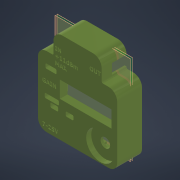
# Autodesk Inventor part: shell
Saved by Autodesk Inventor 2022 (Build 260153000, 153)
## iProperties
Created: 2021-12-11
Part Number: shell
Material: ABS Plastic
Document SubType Name: Modeling
Designer: nebst
Density: 1.06 g/cm^3
Appearance: Dark Olive
Author: nebst
Autodesk Inventor part; units mm, degrees
(part 1 of 2)
ref_plane "YZ Plane" through (0, 0, 0) normal (1, 0, 0) x (0, 1, 0)
ref_plane "XZ Plane" through (0, 0, 0) normal (0, 1, 0) x (-1, 0, 0)
ref_plane "XY Plane" through (0, 0, 0) normal (0, 0, 1) x (1, 0, 0)
ref_plane "board backside" through (0, 0, -1.6) normal (0, 0, -1) x (-1, 0, 0)
sketch "Sketch1" plane through (0, 0, -1.6) normal (0, 0, -1) x (-1, 0, 0)
  line L0 (-26.924, -27.6401) -> (-26.924, 15.0319) projected
  arc A0 (-26.924, -27.6401) -> (-24.384, -30.1801) centre (-24.384, -27.6401) ccw projected
  line L1 (24.384, -30.1801) -> (-24.384, -30.1801) projected
  arc A1 (24.384, -30.1801) -> (26.924, -27.6401) centre (24.384, -27.6401) ccw projected
  line L2 (26.924, 16.5559) -> (26.924, -27.6401) projected
  arc A2 (26.924, 16.5559) -> (24.384, 19.0959) centre (24.384, 16.5559) ccw projected
  line L3 (19.812, 19.0959) -> (24.384, 19.0959) projected
  arc A3 (17.272, 21.6359) -> (19.812, 19.0959) centre (19.812, 21.6359) ccw projected
  line L4 (17.272, 30.7799) -> (17.272, 21.6359) projected
  arc A4 (17.272, 30.7799) -> (14.732, 33.3199) centre (14.732, 30.7799) ccw projected
  line L5 (-14.732, 33.3199) -> (14.732, 33.3199) projected
  arc A5 (-14.732, 33.3199) -> (-17.272, 30.7799) centre (-14.732, 30.7799) ccw projected
  line L6 (-17.272, 21.6359) -> (-17.272, 30.7799) projected
  arc A6 (-19.812, 19.0959) -> (-17.272, 21.6359) centre (-19.812, 21.6359) ccw projected
  line L7 (-24.384, 19.0959) -> (-19.812, 19.0959) projected
  arc A7 (-24.384, 19.0959) -> (-26.924, 16.5559) centre (-24.384, 16.5559) ccw projected
  line L8 (-26.924, 15.0319) -> (-26.924, 16.5559) projected
  line L9 (20.978, -21.5601) -> (20.978, -23.5601) projected
  arc A8 (19.978, -23.5601) -> (20.978, -23.5601) centre (20.478, -23.5601) ccw projected
  line L10 (19.978, -23.5601) -> (19.978, -21.5601) projected
  arc A9 (20.978, -21.5601) -> (19.978, -21.5601) centre (20.478, -21.5601) ccw projected
  line L11 (16.478, -26.7601) -> (18.478, -26.7601) projected
  arc A10 (18.478, -27.7601) -> (18.478, -26.7601) centre (18.478, -27.2601) ccw projected
  line L12 (18.478, -27.7601) -> (16.478, -27.7601) projected
  arc A11 (16.478, -26.7601) -> (16.478, -27.7601) centre (16.478, -27.2601) ccw projected
  line L13 (14.978, -21.5601) -> (14.978, -23.5601) projected
  arc A12 (13.978, -23.5601) -> (14.978, -23.5601) centre (14.478, -23.5601) ccw projected
  line L14 (13.978, -23.5601) -> (13.978, -21.5601) projected
  arc A13 (14.978, -21.5601) -> (13.978, -21.5601) centre (14.478, -21.5601) ccw projected
  circle A14 centre (19.558, -14.3051) radius 0.5 projected
  circle A15 centre (24.003, -9.8601) radius 0.5 projected
  circle A16 centre (21.463, -9.8601) radius 0.5 projected
  circle A17 centre (18.923, -9.8601) radius 0.5 projected
  circle A18 centre (17.018, -14.3051) radius 0.5 projected
  circle A19 centre (16.383, -9.8601) radius 0.5 projected
  circle A20 centre (7.493, -14.3051) radius 0.5 projected
  circle A21 centre (4.953, -14.3051) radius 0.5 projected
  circle A22 centre (10.922, -1.2241) radius 0.5 projected
  circle A23 centre (8.382, -1.2241) radius 0.5 projected
  circle A24 centre (2.54, -5.0341) radius 0.35 projected
  circle A25 centre (0, -5.0341) radius 0.35 projected
  circle A26 centre (-10.287, -25.0201) radius 0.5 projected
  circle A27 centre (-10.287, -22.5201) radius 0.5 projected
  circle A28 centre (-10.287, -20.0201) radius 0.5 projected
  circle A29 centre (-17.787, -28.1201) radius 1.3 projected
  circle A30 centre (-24.787, -25.0201) radius 0.5 projected
  circle A31 centre (-17.787, -16.9201) radius 1.3 projected
  circle A32 centre (-24.787, -20.0201) radius 0.5 projected
  circle A33 centre (-2.54, -5.0341) radius 0.35 projected
  circle A34 centre (-5.08, -5.0341) radius 0.35 projected
  circle A35 centre (-7.62, -5.0341) radius 0.35 projected
  circle A36 centre (-10.16, -5.0341) radius 0.35 projected
  circle A37 centre (-12.7, -5.0341) radius 0.35 projected
  circle A38 centre (-15.24, -5.0341) radius 0.35 projected
  circle A39 centre (23.368, 10.4599) radius 0.5 projected
  circle A40 centre (20.828, 10.4599) radius 0.5 projected
  circle A41 centre (18.288, 10.4599) radius 0.5 projected
  circle A42 centre (10.922, 1.3159) radius 0.5 projected
  circle A43 centre (8.382, 1.3159) radius 0.5 projected
  circle A44 centre (10.922, 3.8559) radius 0.5 projected
  circle A45 centre (10.922, 6.3959) radius 0.5 projected
  circle A46 centre (8.382, 3.8559) radius 0.5 projected
  circle A47 centre (8.382, 6.3959) radius 0.5 projected
  circle A48 centre (2.54, 5.1259) radius 0.35 projected
  circle A49 centre (0, 5.1259) radius 0.35 projected
  circle A50 centre (16.818, 23.0329) radius 0.1 projected
  circle A51 centre (16.818, 23.6679) radius 0.1 projected
  circle A52 centre (16.31, 23.0329) radius 0.1 projected
  circle A53 centre (15.802, 23.0329) radius 0.1 projected
  circle A54 centre (15.294, 23.0329) radius 0.1 projected
  circle A55 centre (16.31, 23.6679) radius 0.1 projected
  circle A56 centre (15.802, 23.6679) radius 0.1 projected
  circle A57 centre (15.294, 23.6679) radius 0.1 projected
  circle A58 centre (14.786, 23.0329) radius 0.1 projected
  circle A59 centre (14.278, 23.0329) radius 0.1 projected
  circle A60 centre (13.77, 23.0329) radius 0.1 projected
  circle A61 centre (14.786, 23.6679) radius 0.1 projected
  circle A62 centre (14.278, 23.6679) radius 0.1 projected
  circle A63 centre (13.77, 23.6679) radius 0.1 projected
  circle A64 centre (13.262, 23.0329) radius 0.1 projected
  circle A65 centre (13.262, 23.6679) radius 0.1 projected
  circle A66 centre (16.818, 28.7479) radius 0.1 projected
  circle A67 centre (16.818, 29.3829) radius 0.1 projected
  circle A68 centre (16.31, 28.7479) radius 0.1 projected
  circle A69 centre (16.31, 29.3829) radius 0.1 projected
  circle A70 centre (15.802, 28.7479) radius 0.1 projected
  circle A71 centre (15.294, 28.7479) radius 0.1 projected
  circle A72 centre (15.802, 29.3829) radius 0.1 projected
  circle A73 centre (15.294, 29.3829) radius 0.1 projected
  circle A74 centre (14.786, 28.7479) radius 0.1 projected
  circle A75 centre (14.786, 29.3829) radius 0.1 projected
  circle A76 centre (14.278, 28.7479) radius 0.1 projected
  circle A77 centre (13.77, 28.7479) radius 0.1 projected
  circle A78 centre (14.278, 29.3829) radius 0.1 projected
  circle A79 centre (13.77, 29.3829) radius 0.1 projected
  circle A80 centre (13.262, 28.7479) radius 0.1 projected
  circle A81 centre (13.262, 29.3829) radius 0.1 projected
  circle A82 centre (1.508, 24.9539) radius 0.1 projected
  circle A83 centre (0.508, 24.9539) radius 0.1 projected
  circle A84 centre (1.508, 25.9539) radius 0.1 projected
  circle A85 centre (1.508, 26.9539) radius 0.1 projected
  circle A86 centre (0.508, 25.9539) radius 0.1 projected
  circle A87 centre (0.508, 26.9539) radius 0.1 projected
  circle A88 centre (-2.54, 5.1259) radius 0.35 projected
  circle A89 centre (-5.08, 5.1259) radius 0.35 projected
  circle A90 centre (-7.62, 5.1259) radius 0.35 projected
  circle A91 centre (-10.16, 5.1259) radius 0.35 projected
  circle A92 centre (-12.7, 5.1259) radius 0.35 projected
  circle A93 centre (-15.24, 5.1259) radius 0.35 projected
  circle A94 centre (-0.492, 24.9539) radius 0.1 projected
  circle A95 centre (-0.492, 25.9539) radius 0.1 projected
  circle A96 centre (-0.492, 26.9539) radius 0.1 projected
  circle A97 centre (-13.462, 23.0329) radius 0.1 projected
  circle A98 centre (-13.97, 23.0329) radius 0.1 projected
  circle A99 centre (-13.462, 23.6679) radius 0.1 projected
  circle A100 centre (-13.97, 23.6679) radius 0.1 projected
  circle A101 centre (-14.478, 23.0329) radius 0.1 projected
  circle A102 centre (-14.986, 23.0329) radius 0.1 projected
  circle A103 centre (-15.494, 23.0329) radius 0.1 projected
  circle A104 centre (-14.478, 23.6679) radius 0.1 projected
  circle A105 centre (-14.986, 23.6679) radius 0.1 projected
  circle A106 centre (-15.494, 23.6679) radius 0.1 projected
  circle A107 centre (-16.002, 23.0329) radius 0.1 projected
  circle A108 centre (-16.51, 23.0329) radius 0.1 projected
  circle A109 centre (-17.018, 23.0329) radius 0.1 projected
  circle A110 centre (-16.002, 23.6679) radius 0.1 projected
  circle A111 centre (-16.51, 23.6679) radius 0.1 projected
  circle A112 centre (-17.018, 23.6679) radius 0.1 projected
  circle A113 centre (-13.462, 28.7479) radius 0.1 projected
  circle A114 centre (-13.462, 29.3829) radius 0.1 projected
  circle A115 centre (-13.97, 28.7479) radius 0.1 projected
  circle A116 centre (-13.97, 29.3829) radius 0.1 projected
  circle A117 centre (-14.478, 28.7479) radius 0.1 projected
  circle A118 centre (-14.986, 28.7479) radius 0.1 projected
  circle A119 centre (-14.478, 29.3829) radius 0.1 projected
  circle A120 centre (-14.986, 29.3829) radius 0.1 projected
  circle A121 centre (-15.494, 28.7479) radius 0.1 projected
  circle A122 centre (-15.494, 29.3829) radius 0.1 projected
  circle A123 centre (-16.002, 28.7479) radius 0.1 projected
  circle A124 centre (-16.51, 28.7479) radius 0.1 projected
  circle A125 centre (-16.002, 29.3829) radius 0.1 projected
  circle A126 centre (-16.51, 29.3829) radius 0.1 projected
  circle A127 centre (-17.018, 28.7479) radius 0.1 projected
  circle A128 centre (-17.018, 29.3829) radius 0.1 projected
  line L15 (-27.074, 15.0319) -> (-27.074, -27.6401)
  arc A129 (-27.074, -27.6401) -> (-24.384, -30.3301) centre (-24.384, -27.6401) ccw
  line L16 (-24.384, -30.3301) -> (24.384, -30.3301)
  arc A130 (24.384, -30.3301) -> (27.074, -27.6401) centre (24.384, -27.6401) ccw
  line L17 (27.074, -27.6401) -> (27.074, 16.5559)
  arc A131 (27.074, 16.5559) -> (24.384, 19.2459) centre (24.384, 16.5559) ccw
  line L18 (24.384, 19.2459) -> (19.812, 19.2459)
  arc A132 (17.422, 21.6359) -> (19.812, 19.2459) centre (19.812, 21.6359) ccw
  line L19 (17.422, 21.6359) -> (17.422, 30.7799)
  arc A133 (17.422, 30.7799) -> (14.732, 33.4699) centre (14.732, 30.7799) ccw
  line L20 (14.732, 33.4699) -> (-14.732, 33.4699)
  arc A134 (-14.732, 33.4699) -> (-17.422, 30.7799) centre (-14.732, 30.7799) ccw
  line L21 (-17.422, 30.7799) -> (-17.422, 21.6359)
  arc A135 (-19.812, 19.2459) -> (-17.422, 21.6359) centre (-19.812, 21.6359) ccw
  line L22 (-19.812, 19.2459) -> (-24.384, 19.2459)
  arc A136 (-24.384, 19.2459) -> (-27.074, 16.5559) centre (-24.384, 16.5559) ccw
  line L23 (-27.074, 16.5559) -> (-27.074, 15.0319)
  line L24 (31.074, 13.9559) -> (31.074, -27.6401)
  arc A137 (24.384, -34.3301) -> (31.074, -27.6401) centre (24.384, -27.6401) ccw
  line L25 (24.384, -34.3301) -> (-24.384, -34.3301)
  arc A138 (-31.074, -27.6401) -> (-24.384, -34.3301) centre (-24.384, -27.6401) ccw
  line L26 (-31.074, -27.6401) -> (-31.074, 13.9559)
  line L27 (-18.922, 21.7459) -> (-18.922, 30.6799)
  line L28 (-12.132, 37.4699) -> (12.132, 37.4699)
  line L29 (18.922, 30.6799) -> (18.922, 21.7459)
  line L30 (19.922, 20.7459) -> (24.284, 20.7459)
  line L31 (-24.284, 20.7459) -> (-19.922, 20.7459)
  arc A139 (-24.284, 20.7459) -> (-31.074, 13.9559) centre (-24.284, 13.9559) ccw
  arc A140 (31.074, 13.9559) -> (24.284, 20.7459) centre (24.284, 13.9559) ccw
  arc A141 (-19.922, 20.7459) -> (-18.922, 21.7459) centre (-19.922, 21.7459) ccw
  arc A142 (18.922, 21.7459) -> (19.922, 20.7459) centre (19.922, 21.7459) ccw
  arc A143 (18.922, 30.6799) -> (12.132, 37.4699) centre (12.132, 30.6799) ccw
  arc A144 (-12.132, 37.4699) -> (-18.922, 30.6799) centre (-12.132, 30.6799) ccw
  point P0 (0, 0)
  dimension "d0" = 0.15
  dimension "d3" = 6.79
  dimension "d4" = 4
  dimension "d5" = 4
  dimension "d6" = 1
  dimension "d7" = 1.5
  dimension "d8" = 1.5
  dimension "d9" = 1.5
  dimension "d10" = 1.5
  dimension "d11" = 6.79
  constraints: 34 end point, 32 point on circle, 16 centre point, 12 tangent, 3 equal radius, 20 other
  measures "d0" distance between parallel lines of L0 L15
  measures "d3" radius of A139
  measures "d4" distance between parallel lines of L20 L28
  measures "d5" distance between parallel lines of L26 L15
  measures "d6" radius of A141
  measures "d7" distance between parallel lines of L18 L30
  measures "d8" distance between parallel lines of L22 L31
  measures "d9" distance between parallel lines of L21 L27
  measures "d10" distance between parallel lines of L19 L29
  measures "d11" radius of A143
extrude "side walls" add sketch "Sketch1" against normal blind 13.5 contours L24 A137 L25 A138 L26 A139 L31 A141 L27 A144 L28 A143 L29 A142 L30 A140
sketch "Sketch2" plane through (0, 0, 11.9) normal (0, 0, 1) x (1, 0, 0)
  line L0 (12.132, 37.4699) -> (-12.132, 37.4699)
  arc A0 (-12.132, 37.4699) -> (-18.922, 30.6799) centre (-12.132, 30.6799) ccw
  line L1 (-18.922, 30.6799) -> (-18.922, 21.7459)
  arc A1 (-19.922, 20.7459) -> (-18.922, 21.7459) centre (-19.922, 21.7459) ccw
  line L2 (-19.922, 20.7459) -> (-24.284, 20.7459)
  arc A2 (-24.284, 20.7459) -> (-31.074, 13.9559) centre (-24.284, 13.9559) ccw
  line L3 (-31.074, 13.9559) -> (-31.074, -27.6401)
  arc A3 (-31.074, -27.6401) -> (-24.384, -34.3301) centre (-24.384, -27.6401) ccw
  line L4 (-24.384, -34.3301) -> (24.384, -34.3301)
  arc A4 (24.384, -34.3301) -> (31.074, -27.6401) centre (24.384, -27.6401) ccw
  line L5 (31.074, -27.6401) -> (31.074, 13.9559)
  arc A5 (31.074, 13.9559) -> (24.284, 20.7459) centre (24.284, 13.9559) ccw
  line L6 (24.284, 20.7459) -> (19.922, 20.7459)
  arc A6 (18.922, 21.7459) -> (19.922, 20.7459) centre (19.922, 21.7459) ccw
  line L7 (18.922, 21.7459) -> (18.922, 30.6799)
  arc A7 (18.922, 30.6799) -> (12.132, 37.4699) centre (12.132, 30.6799) ccw
  arc A8 (17.422, 21.6359) -> (19.812, 19.2459) centre (19.812, 21.6359) ccw
  line L8 (19.812, 19.2459) -> (24.384, 19.2459)
  arc A9 (27.074, 16.5559) -> (24.384, 19.2459) centre (24.384, 16.5559) ccw
  line L9 (27.074, 16.5559) -> (27.074, -27.6401)
  arc A10 (24.384, -30.3301) -> (27.074, -27.6401) centre (24.384, -27.6401) ccw
  line L10 (24.384, -30.3301) -> (-24.384, -30.3301)
  arc A11 (-27.074, -27.6401) -> (-24.384, -30.3301) centre (-24.384, -27.6401) ccw
  line L11 (-27.074, -27.6401) -> (-27.074, 16.5559)
  arc A12 (-24.384, 19.2459) -> (-27.074, 16.5559) centre (-24.384, 16.5559) ccw
  line L12 (-24.384, 19.2459) -> (-19.812, 19.2459)
  arc A13 (-19.812, 19.2459) -> (-17.422, 21.6359) centre (-19.812, 21.6359) ccw
  line L13 (-17.422, 21.6359) -> (-17.422, 30.7799)
  arc A14 (-14.732, 33.4699) -> (-17.422, 30.7799) centre (-14.732, 30.7799) ccw
  line L14 (-14.732, 33.4699) -> (14.732, 33.4699)
  arc A15 (17.422, 30.7799) -> (14.732, 33.4699) centre (14.732, 30.7799) ccw
  line L15 (17.422, 30.7799) -> (17.422, 21.6359)
  line L16 (-24.638, 9.4439) -> (-24.384, 9.1899)
  line L17 (-24.384, 9.1899) -> (-22.352, 9.1899)
  line L18 (-22.352, 9.1899) -> (-22.098, 9.4439)
  line L19 (-22.098, 9.4439) -> (-21.844, 9.1899)
  line L20 (-21.844, 9.1899) -> (-19.812, 9.1899)
  line L21 (-19.812, 9.1899) -> (-19.558, 9.4439)
  line L22 (-19.558, 9.4439) -> (-19.304, 9.1899)
  line L23 (-19.304, 9.1899) -> (-17.272, 9.1899)
  line L24 (-17.272, 9.1899) -> (-17.018, 9.4439)
  line L25 (-17.018, 9.4439) -> (-17.018, 11.4759)
  line L26 (-17.018, 11.4759) -> (-17.272, 11.7299)
  line L27 (-17.272, 11.7299) -> (-19.304, 11.7299)
  line L28 (-19.304, 11.7299) -> (-19.558, 11.4759)
  line L29 (-19.558, 11.4759) -> (-19.812, 11.7299)
  line L30 (-19.812, 11.7299) -> (-21.844, 11.7299)
  line L31 (-21.844, 11.7299) -> (-22.098, 11.4759)
  line L32 (-22.098, 11.4759) -> (-22.352, 11.7299)
  line L33 (-22.352, 11.7299) -> (-24.384, 11.7299)
  line L34 (-24.384, 11.7299) -> (-24.638, 11.4759)
  line L35 (-24.638, 11.4759) -> (-24.638, 9.4439)
  line L36 (-23.048, 10.7799) -> (-23.688, 10.7799)
  line L37 (-23.048, 10.7799) -> (-23.048, 10.1399)
  line L38 (-23.048, 10.1399) -> (-23.688, 10.1399)
  line L39 (-23.688, 10.7799) -> (-23.688, 10.1399)
  line L40 (-20.508, 10.7799) -> (-20.508, 10.1399)
  line L41 (-20.508, 10.1399) -> (-21.148, 10.1399)
  line L42 (-21.148, 10.7799) -> (-21.148, 10.1399)
  line L43 (-20.508, 10.7799) -> (-21.148, 10.7799)
  line L44 (-18.608, 10.7799) -> (-18.608, 10.1399)
  line L45 (-17.968, 10.7799) -> (-18.608, 10.7799)
  line L46 (-17.968, 10.7799) -> (-17.968, 10.1399)
  line L47 (-17.968, 10.1399) -> (-18.608, 10.1399)
  line L48 (-15.113, -8.8441) -> (-15.367, -8.5901)
  line L49 (-15.367, -8.5901) -> (-17.399, -8.5901)
  line L50 (-17.399, -8.5901) -> (-17.653, -8.8441)
  line L51 (-17.653, -8.8441) -> (-17.907, -8.5901)
  line L52 (-17.907, -8.5901) -> (-19.939, -8.5901)
  line L53 (-19.939, -8.5901) -> (-20.193, -8.8441)
  line L54 (-20.193, -8.8441) -> (-20.447, -8.5901)
  line L55 (-20.447, -8.5901) -> (-22.479, -8.5901)
  line L56 (-22.479, -8.5901) -> (-22.733, -8.8441)
  line L57 (-22.733, -8.8441) -> (-22.987, -8.5901)
  line L58 (-22.987, -8.5901) -> (-25.019, -8.5901)
  line L59 (-25.019, -8.5901) -> (-25.273, -8.8441)
  line L60 (-25.273, -8.8441) -> (-25.273, -10.8761)
  line L61 (-25.273, -10.8761) -> (-25.019, -11.1301)
  line L62 (-25.019, -11.1301) -> (-22.987, -11.1301)
  line L63 (-22.987, -11.1301) -> (-22.733, -10.8761)
  line L64 (-22.733, -10.8761) -> (-22.479, -11.1301)
  line L65 (-22.479, -11.1301) -> (-20.447, -11.1301)
  line L66 (-20.447, -11.1301) -> (-20.193, -10.8761)
  line L67 (-20.193, -10.8761) -> (-19.939, -11.1301)
  line L68 (-19.939, -11.1301) -> (-17.907, -11.1301)
  line L69 (-17.907, -11.1301) -> (-17.653, -10.8761)
  line L70 (-17.653, -10.8761) -> (-17.399, -11.1301)
  line L71 (-17.399, -11.1301) -> (-15.367, -11.1301)
  line L72 (-15.367, -11.1301) -> (-15.113, -10.8761)
  line L73 (-15.113, -10.8761) -> (-15.113, -8.8441)
  line L74 (-21.143, -10.1801) -> (-21.143, -9.5401)
  line L75 (-21.783, -10.1801) -> (-21.143, -10.1801)
  line L76 (-21.783, -10.1801) -> (-21.783, -9.5401)
  line L77 (-21.783, -9.5401) -> (-21.143, -9.5401)
  line L78 (-24.323, -10.1801) -> (-23.683, -10.1801)
  line L79 (-24.323, -10.1801) -> (-24.323, -9.5401)
  line L80 (-24.323, -9.5401) -> (-23.683, -9.5401)
  line L81 (-23.683, -10.1801) -> (-23.683, -9.5401)
  line L82 (-16.703, -10.1801) -> (-16.063, -10.1801)
  line L83 (-16.703, -10.1801) -> (-16.703, -9.5401)
  line L84 (-16.703, -9.5401) -> (-16.063, -9.5401)
  line L85 (-16.063, -10.1801) -> (-16.063, -9.5401)
  line L86 (-18.603, -10.1801) -> (-18.603, -9.5401)
  line L87 (-19.243, -10.1801) -> (-18.603, -10.1801)
  line L88 (-19.243, -10.1801) -> (-19.243, -9.5401)
  line L89 (-19.243, -9.5401) -> (-18.603, -9.5401)
  line L90 (-15.748, -13.2891) -> (-16.002, -13.0351)
  line L91 (-16.002, -13.0351) -> (-18.034, -13.0351)
  line L92 (-18.034, -13.0351) -> (-18.288, -13.2891)
  line L93 (-18.288, -13.2891) -> (-18.542, -13.0351)
  line L94 (-18.542, -13.0351) -> (-20.574, -13.0351)
  line L95 (-20.574, -13.0351) -> (-20.828, -13.2891)
  line L96 (-20.828, -13.2891) -> (-20.828, -15.3211)
  line L97 (-20.828, -15.3211) -> (-20.574, -15.5751)
  line L98 (-20.574, -15.5751) -> (-18.542, -15.5751)
  line L99 (-18.542, -15.5751) -> (-18.288, -15.3211)
  line L100 (-18.288, -15.3211) -> (-18.034, -15.5751)
  line L101 (-18.034, -15.5751) -> (-16.002, -15.5751)
  line L102 (-16.002, -15.5751) -> (-15.748, -15.3211)
  line L103 (-15.748, -15.3211) -> (-15.748, -13.2891)
  line L104 (-17.338, -14.6251) -> (-17.338, -13.9851)
  line L105 (-17.338, -13.9851) -> (-16.698, -13.9851)
  line L106 (-16.698, -14.6251) -> (-16.698, -13.9851)
  line L107 (-17.338, -14.6251) -> (-16.698, -14.6251)
  line L108 (-19.878, -14.6251) -> (-19.878, -13.9851)
  line L109 (-19.878, -13.9851) -> (-19.238, -13.9851)
  line L110 (-19.238, -14.6251) -> (-19.238, -13.9851)
  line L111 (-19.878, -14.6251) -> (-19.238, -14.6251)
  line L112 (-3.683, -13.2891) -> (-3.937, -13.0351)
  line L113 (-3.937, -13.0351) -> (-5.969, -13.0351)
  line L114 (-5.969, -13.0351) -> (-6.223, -13.2891)
  line L115 (-6.223, -13.2891) -> (-6.477, -13.0351)
  line L116 (-6.477, -13.0351) -> (-8.509, -13.0351)
  line L117 (-8.509, -13.0351) -> (-8.763, -13.2891)
  line L118 (-8.763, -13.2891) -> (-8.763, -15.3211)
  line L119 (-8.763, -15.3211) -> (-8.509, -15.5751)
  line L120 (-8.509, -15.5751) -> (-6.477, -15.5751)
  line L121 (-6.477, -15.5751) -> (-6.223, -15.3211)
  line L122 (-6.223, -15.3211) -> (-5.969, -15.5751)
  line L123 (-5.969, -15.5751) -> (-3.937, -15.5751)
  line L124 (-3.937, -15.5751) -> (-3.683, -15.3211)
  line L125 (-3.683, -15.3211) -> (-3.683, -13.2891)
  line L126 (-5.273, -14.6251) -> (-5.273, -13.9851)
  line L127 (-5.273, -13.9851) -> (-4.633, -13.9851)
  line L128 (-4.633, -14.6251) -> (-4.633, -13.9851)
  line L129 (-5.273, -14.6251) -> (-4.633, -14.6251)
  line L130 (-7.813, -14.6251) -> (-7.813, -13.9851)
  line L131 (-7.813, -13.9851) -> (-7.173, -13.9851)
  line L132 (-7.173, -14.6251) -> (-7.173, -13.9851)
  line L133 (-7.813, -14.6251) -> (-7.173, -14.6251)
  line L134 (26.4, -6.3041) -> (26.4, 6.3959)
  line L135 (26.4, 6.3959) -> (-13.7, 6.3959)
  line L136 (-13.7, 6.3959) -> (-13.7, -6.3041)
  line L137 (-13.7, -6.3041) -> (26.4, -6.3041)
  line L138 (20.3476, 4.1754) -> (19.9121, 4.7197)
  line L139 (19.9121, 4.7197) -> (20.3014, 5.0311)
  line L140 (20.3014, 5.0311) -> (24.5951, 5.0464)
  line L141 (24.5951, 5.0464) -> (24.8689, 4.7041)
  line L142 (24.8689, 4.7041) -> (24.208, 4.1754)
  line L143 (24.208, 4.1754) -> (20.3476, 4.1754)
  line L144 (24.6494, 0.1774) -> (23.8633, 0.6371)
  line L145 (23.8633, 0.6371) -> (24.387, 3.897)
  line L146 (24.387, 3.897) -> (25.052, 4.4753)
  line L147 (25.052, 4.4753) -> (25.2917, 4.1756)
  line L148 (25.2917, 4.1756) -> (24.6494, 0.1774)
  line L149 (19.3167, -0.5453) -> (18.793, -3.8051)
  line L150 (18.793, -3.8051) -> (18.128, -4.3835)
  line L151 (18.128, -4.3835) -> (17.8883, -4.0838)
  line L152 (17.8883, -4.0838) -> (18.5306, -0.0855)
  line L153 (18.5306, -0.0855) -> (19.3167, -0.5453)
  line L154 (23.2679, -4.6279) -> (22.8786, -4.9393)
  line L155 (22.8786, -4.9393) -> (18.5849, -4.9546)
  line L156 (18.5849, -4.9546) -> (18.3111, -4.6123)
  line L157 (18.3111, -4.6123) -> (18.972, -4.0835)
  line L158 (18.972, -4.0835) -> (22.8324, -4.0835)
  line L159 (22.8324, -4.0835) -> (23.2679, -4.6279)
  line L160 (14.892, 4.4753) -> (15.1317, 4.1756)
  line L161 (15.1317, 4.1756) -> (14.4894, 0.1774)
  line L162 (14.4894, 0.1774) -> (13.7033, 0.6371)
  line L163 (13.7033, 0.6371) -> (14.227, 3.897)
  line L164 (14.227, 3.897) -> (14.892, 4.4753)
  line L165 (12.6724, -4.0835) -> (13.1079, -4.6279)
  line L166 (13.1079, -4.6279) -> (12.7186, -4.9393)
  line L167 (12.7186, -4.9393) -> (8.4249, -4.9546)
  line L168 (8.4249, -4.9546) -> (8.1511, -4.6123)
  line L169 (8.1511, -4.6123) -> (8.812, -4.0835)
  line L170 (8.812, -4.0835) -> (12.6724, -4.0835)
  line L171 (8.3706, -0.0855) -> (9.1567, -0.5453)
  line L172 (9.1567, -0.5453) -> (8.633, -3.8051)
  line L173 (8.633, -3.8051) -> (7.968, -4.3835)
  line L174 (7.968, -4.3835) -> (7.7283, -4.0838)
  line L175 (7.7283, -4.0838) -> (8.3706, -0.0855)
  line L176 (14.7089, 4.7041) -> (14.048, 4.1754)
  line L177 (14.048, 4.1754) -> (10.1876, 4.1754)
  line L178 (10.1876, 4.1754) -> (9.7521, 4.7197)
  line L179 (9.7521, 4.7197) -> (10.1414, 5.0311)
  line L180 (10.1414, 5.0311) -> (14.4351, 5.0464)
  line L181 (14.4351, 5.0464) -> (14.7089, 4.7041)
  line L182 (4.732, 4.4753) -> (4.9717, 4.1756)
  line L183 (4.9717, 4.1756) -> (4.3294, 0.1774)
  line L184 (4.3294, 0.1774) -> (3.5433, 0.6371)
  line L185 (3.5433, 0.6371) -> (4.067, 3.897)
  line L186 (4.067, 3.897) -> (4.732, 4.4753)
  line L187 (2.5124, -4.0835) -> (2.9479, -4.6279)
  line L188 (2.9479, -4.6279) -> (2.5586, -4.9393)
  line L189 (2.5586, -4.9393) -> (-1.7351, -4.9546)
  line L190 (-1.7351, -4.9546) -> (-2.0089, -4.6123)
  line L191 (-2.0089, -4.6123) -> (-1.348, -4.0835)
  line L192 (-1.348, -4.0835) -> (2.5124, -4.0835)
  line L193 (-1.7894, -0.0855) -> (-1.0033, -0.5453)
  line L194 (-1.0033, -0.5453) -> (-1.527, -3.8051)
  line L195 (-1.527, -3.8051) -> (-2.192, -4.3835)
  line L196 (-2.192, -4.3835) -> (-2.4317, -4.0838)
  line L197 (-2.4317, -4.0838) -> (-1.7894, -0.0855)
  line L198 (4.5489, 4.7041) -> (3.888, 4.1754)
  line L199 (3.888, 4.1754) -> (0.0276, 4.1754)
  line L200 (0.0276, 4.1754) -> (-0.4079, 4.7197)
  line L201 (-0.4079, 4.7197) -> (-0.0186, 5.0311)
  line L202 (-0.0186, 5.0311) -> (4.2751, 5.0464)
  line L203 (4.2751, 5.0464) -> (4.5489, 4.7041)
  line L204 (-7.6476, -4.0835) -> (-7.2121, -4.6279)
  line L205 (-7.2121, -4.6279) -> (-7.6014, -4.9393)
  line L206 (-7.6014, -4.9393) -> (-11.8951, -4.9546)
  line L207 (-11.8951, -4.9546) -> (-12.1689, -4.6123)
  line L208 (-12.1689, -4.6123) -> (-11.508, -4.0835)
  line L209 (-11.508, -4.0835) -> (-7.6476, -4.0835)
  line L210 (-5.428, 4.4753) -> (-5.1883, 4.1756)
  line L211 (-5.1883, 4.1756) -> (-5.8306, 0.1774)
  line L212 (-5.8306, 0.1774) -> (-6.6167, 0.6371)
  line L213 (-6.6167, 0.6371) -> (-6.093, 3.897)
  line L214 (-6.093, 3.897) -> (-5.428, 4.4753)
  line L215 (-5.6111, 4.7041) -> (-6.272, 4.1754)
  line L216 (-6.272, 4.1754) -> (-10.1324, 4.1754)
  line L217 (-10.1324, 4.1754) -> (-10.5679, 4.7197)
  line L218 (-10.5679, 4.7197) -> (-10.1786, 5.0311)
  line L219 (-10.1786, 5.0311) -> (-5.8849, 5.0464)
  line L220 (-5.8849, 5.0464) -> (-5.6111, 4.7041)
  line L221 (-11.9494, -0.0855) -> (-11.1633, -0.5453)
  line L222 (-11.1633, -0.5453) -> (-11.687, -3.8051)
  line L223 (-11.687, -3.8051) -> (-12.352, -4.3835)
  line L224 (-12.352, -4.3835) -> (-12.5917, -4.0838)
  line L225 (-12.5917, -4.0838) -> (-11.9494, -0.0855)
  circle A16 centre (-5.5899, -4.3761) radius 0.6
  circle A17 centre (4.5701, -4.3761) radius 0.6
  circle A18 centre (14.7301, -4.3761) radius 0.6
  circle A19 centre (24.8901, -4.3761) radius 0.6
  circle A20 centre (5.9297, -2.4744) radius 0.6
  circle A21 centre (6.8216, 2.5384) radius 0.6
  circle A22 centre (17.784, 4.4351) radius 0.6221
  line L226 (-10.3651, 3.975) -> (-10.8347, 4.4753)
  line L227 (-10.9279, 0.6371) -> (-10.3651, 3.975)
  line L228 (-11.9471, 0.1774) -> (-10.9279, 0.6371)
  line L229 (-11.2468, 4.0885) -> (-11.9471, 0.1774)
  line L230 (-10.8347, 4.4753) -> (-11.2468, 4.0885)
  line L231 (-7.1965, -0.4291) -> (-6.2226, 0.0459)
  line L232 (-10.6853, -0.4291) -> (-7.1965, -0.4291)
  line L233 (-11.508, 0.0459) -> (-10.6853, -0.4291)
  line L234 (-11.508, 0.0459) -> (-10.5341, 0.5209)
  line L235 (-6.9453, 0.5209) -> (-10.5341, 0.5209)
  line L236 (-6.2226, 0.0459) -> (-6.9453, 0.5209)
  line L237 (-6.5332, -3.9967) -> (-5.8329, -0.0855)
  line L238 (-6.9453, -4.3835) -> (-6.5332, -3.9967)
  line L239 (-7.4149, -3.8831) -> (-6.9453, -4.3835)
  line L240 (-6.8521, -0.5453) -> (-7.4149, -3.8831)
  line L241 (-5.8329, -0.0855) -> (-6.8521, -0.5453)
  line L242 (2.9635, -0.4291) -> (3.9374, 0.0459)
  line L243 (-0.5253, -0.4291) -> (2.9635, -0.4291)
  line L244 (-1.348, 0.0459) -> (-0.5253, -0.4291)
  line L245 (-1.348, 0.0459) -> (-0.3741, 0.5209)
  line L246 (3.2147, 0.5209) -> (-0.3741, 0.5209)
  line L247 (3.9374, 0.0459) -> (3.2147, 0.5209)
  line L248 (-0.2051, 3.975) -> (-0.6747, 4.4753)
  line L249 (-0.7679, 0.6371) -> (-0.2051, 3.975)
  line L250 (-1.7871, 0.1774) -> (-0.7679, 0.6371)
  line L251 (-1.0868, 4.0885) -> (-1.7871, 0.1774)
  line L252 (-0.6747, 4.4753) -> (-1.0868, 4.0885)
  line L253 (3.6268, -3.9967) -> (4.3271, -0.0855)
  line L254 (3.2147, -4.3835) -> (3.6268, -3.9967)
  line L255 (2.7451, -3.8831) -> (3.2147, -4.3835)
  line L256 (3.3079, -0.5453) -> (2.7451, -3.8831)
  line L257 (4.3271, -0.0855) -> (3.3079, -0.5453)
  line L258 (9.9549, 3.975) -> (9.4853, 4.4753)
  line L259 (9.3921, 0.6371) -> (9.9549, 3.975)
  line L260 (8.3729, 0.1774) -> (9.3921, 0.6371)
  line L261 (9.0732, 4.0885) -> (8.3729, 0.1774)
  line L262 (9.4853, 4.4753) -> (9.0732, 4.0885)
  line L263 (13.7868, -3.9967) -> (14.4871, -0.0855)
  line L264 (13.3747, -4.3835) -> (13.7868, -3.9967)
  line L265 (12.9051, -3.8831) -> (13.3747, -4.3835)
  line L266 (13.4679, -0.5453) -> (12.9051, -3.8831)
  line L267 (14.4871, -0.0855) -> (13.4679, -0.5453)
  line L268 (13.1235, -0.4291) -> (14.0974, 0.0459)
  line L269 (9.6347, -0.4291) -> (13.1235, -0.4291)
  line L270 (8.812, 0.0459) -> (9.6347, -0.4291)
  line L271 (8.812, 0.0459) -> (9.7859, 0.5209)
  line L272 (13.3747, 0.5209) -> (9.7859, 0.5209)
  line L273 (14.0974, 0.0459) -> (13.3747, 0.5209)
  line L274 (19.2332, 4.0885) -> (18.5329, 0.1774)
  line L275 (19.6453, 4.4753) -> (19.2332, 4.0885)
  line L276 (20.1149, 3.975) -> (19.6453, 4.4753)
  line L277 (19.5521, 0.6371) -> (20.1149, 3.975)
  line L278 (18.5329, 0.1774) -> (19.5521, 0.6371)
  line L279 (24.6471, -0.0855) -> (23.6279, -0.5453)
  line L280 (23.9468, -3.9967) -> (24.6471, -0.0855)
  line L281 (23.5347, -4.3835) -> (23.9468, -3.9967)
  line L282 (23.0651, -3.8831) -> (23.5347, -4.3835)
  line L283 (23.6279, -0.5453) -> (23.0651, -3.8831)
  line L284 (24.2574, 0.0459) -> (23.5347, 0.5209)
  line L285 (23.2835, -0.4291) -> (24.2574, 0.0459)
  line L286 (19.7947, -0.4291) -> (23.2835, -0.4291)
  line L287 (18.972, 0.0459) -> (19.7947, -0.4291)
  line L288 (18.972, 0.0459) -> (19.9459, 0.5209)
  line L289 (23.5347, 0.5209) -> (19.9459, 0.5209)
  line L290 (-22.0511, 12.2299) -> (-19.6049, 12.2299)
  line L291 (-19.6049, 12.2299) -> (-19.558, 12.183)
  line L292 (-19.558, 12.183) -> (-19.5111, 12.2299)
  line L293 (-19.5111, 12.2299) -> (-17.0649, 12.2299)
  line L294 (-17.0649, 12.2299) -> (-16.518, 11.683)
  line L295 (-16.518, 11.683) -> (-16.518, 9.2368)
  line L296 (-16.518, 9.2368) -> (-17.0649, 8.6899)
  line L297 (-17.0649, 8.6899) -> (-19.5111, 8.6899)
  line L298 (-19.5111, 8.6899) -> (-19.558, 8.7368)
  line L299 (-19.558, 8.7368) -> (-19.6049, 8.6899)
  line L300 (-19.6049, 8.6899) -> (-22.0511, 8.6899)
  line L301 (-22.0511, 8.6899) -> (-22.098, 8.7368)
  line L302 (-22.098, 8.7368) -> (-22.1449, 8.6899)
  line L303 (-22.1449, 8.6899) -> (-24.5911, 8.6899)
  line L304 (-24.5911, 8.6899) -> (-25.138, 9.2368)
  line L305 (-25.138, 9.2368) -> (-25.138, 11.683)
  line L306 (-25.138, 11.683) -> (-24.5911, 12.2299)
  line L307 (-24.5911, 12.2299) -> (-22.1449, 12.2299)
  line L308 (-22.1449, 12.2299) -> (-22.098, 12.183)
  line L309 (-22.098, 12.183) -> (-22.0511, 12.2299)
  line L310 (-13.9, 6.5959) -> (26.6, 6.5959)
  line L311 (26.6, 6.5959) -> (26.6, -6.5041)
  line L312 (26.6, -6.5041) -> (-13.9, -6.5041)
  line L313 (-13.9, -6.5041) -> (-13.9, 6.5959)
  line L314 (-20.1461, -8.0901) -> (-17.6999, -8.0901)
  line L315 (-17.6999, -8.0901) -> (-17.653, -8.137)
  line L316 (-17.653, -8.137) -> (-17.6061, -8.0901)
  line L317 (-17.6061, -8.0901) -> (-15.1599, -8.0901)
  line L318 (-15.1599, -8.0901) -> (-14.613, -8.637)
  line L319 (-14.613, -8.637) -> (-14.613, -11.0832)
  line L320 (-14.613, -11.0832) -> (-15.1599, -11.6301)
  line L321 (-15.1599, -11.6301) -> (-17.6061, -11.6301)
  line L322 (-17.6061, -11.6301) -> (-17.653, -11.5832)
  line L323 (-17.653, -11.5832) -> (-17.6999, -11.6301)
  line L324 (-17.6999, -11.6301) -> (-20.1461, -11.6301)
  line L325 (-20.1461, -11.6301) -> (-20.193, -11.5832)
  line L326 (-20.193, -11.5832) -> (-20.2399, -11.6301)
  line L327 (-20.2399, -11.6301) -> (-22.6861, -11.6301)
  line L328 (-22.6861, -11.6301) -> (-22.733, -11.5832)
  line L329 (-22.733, -11.5832) -> (-22.7799, -11.6301)
  line L330 (-22.7799, -11.6301) -> (-25.2261, -11.6301)
  line L331 (-25.2261, -11.6301) -> (-25.773, -11.0832)
  line L332 (-25.773, -11.0832) -> (-25.773, -8.637)
  line L333 (-25.773, -8.637) -> (-25.2261, -8.0901)
  line L334 (-25.2261, -8.0901) -> (-22.7799, -8.0901)
  line L335 (-22.7799, -8.0901) -> (-22.733, -8.137)
  line L336 (-22.733, -8.137) -> (-22.6861, -8.0901)
  line L337 (-22.6861, -8.0901) -> (-20.2399, -8.0901)
  line L338 (-20.2399, -8.0901) -> (-20.193, -8.137)
  line L339 (-20.193, -8.137) -> (-20.1461, -8.0901)
  line L340 (-20.7811, -12.5351) -> (-18.3349, -12.5351)
  line L341 (-18.3349, -12.5351) -> (-18.288, -12.582)
  line L342 (-18.288, -12.582) -> (-18.2411, -12.5351)
  line L343 (-18.2411, -12.5351) -> (-15.7949, -12.5351)
  line L344 (-15.7949, -12.5351) -> (-15.248, -13.082)
  line L345 (-15.248, -13.082) -> (-15.248, -15.5282)
  line L346 (-15.248, -15.5282) -> (-15.7949, -16.0751)
  line L347 (-15.7949, -16.0751) -> (-18.2411, -16.0751)
  line L348 (-18.2411, -16.0751) -> (-18.288, -16.0282)
  line L349 (-18.288, -16.0282) -> (-18.3349, -16.0751)
  line L350 (-18.3349, -16.0751) -> (-20.7811, -16.0751)
  line L351 (-20.7811, -16.0751) -> (-21.328, -15.5282)
  line L352 (-21.328, -15.5282) -> (-21.328, -13.082)
  line L353 (-21.328, -13.082) -> (-20.7811, -12.5351)
  line L354 (-8.7161, -12.5351) -> (-6.2699, -12.5351)
  line L355 (-6.2699, -12.5351) -> (-6.223, -12.582)
  line L356 (-6.223, -12.582) -> (-6.1761, -12.5351)
  line L357 (-6.1761, -12.5351) -> (-3.7299, -12.5351)
  line L358 (-3.7299, -12.5351) -> (-3.183, -13.082)
  line L359 (-3.183, -13.082) -> (-3.183, -15.5282)
  line L360 (-3.183, -15.5282) -> (-3.7299, -16.0751)
  line L361 (-3.7299, -16.0751) -> (-6.1761, -16.0751)
  line L362 (-6.1761, -16.0751) -> (-6.223, -16.0282)
  line L363 (-6.223, -16.0282) -> (-6.2699, -16.0751)
  line L364 (-6.2699, -16.0751) -> (-8.7161, -16.0751)
  line L365 (-8.7161, -16.0751) -> (-9.263, -15.5282)
  line L366 (-9.263, -15.5282) -> (-9.263, -13.082)
  line L367 (-9.263, -13.082) -> (-8.7161, -12.5351)
  circle A23 centre (17.787, -22.5201) radius 1.5
  circle A24 centre (17.787, -22.5201) radius 3.75
  point P0 (0, 0)
extrude "front cutouts" add sketch "Sketch2" against normal blind 6 contours A8 L8 A9 L9 A10 L10 A11 L11 A12 L12 A13 L13 A14 L14 A15 L15
sketch "Sketch3" plane through (0, 0, -1.6) normal (0, 0, -1) x (-1, 0, 0)
  line L0 (-9.387, -15.4201) -> (-25.487, -15.4201)
  line L1 (-25.487, -15.4201) -> (-25.487, -26.6701)
  line L2 (-22.487, -29.6701) -> (-9.387, -29.6701)
  line L3 (-9.387, -29.6701) -> (-9.387, -15.4201)
  line L4 (-15.077, -28.4201) -> (-13.287, -28.4201) projected
  line L5 (-13.287, -16.6201) -> (-15.077, -16.6201) projected
  line L6 (-11.787, -18.5201) -> (-11.787, -26.5201) projected
  line L7 (-23.787, -26.5201) -> (-23.787, -18.5201) projected
  line L8 (-20.496, -16.6201) -> (-22.286, -16.6201) projected
  line L9 (-20.496, -28.4201) -> (-22.286, -28.4201) projected
  arc A0 (-25.487, -26.6701) -> (-22.487, -29.6701) centre (-22.487, -26.6701) ccw
  line L10 (13.478, -27.5601) -> (16.478, -27.5601) projected
  line L11 (16.478, -17.5601) -> (13.478, -17.5601) projected
  line L12 (13.478, -17.5601) -> (13.478, -27.5601) projected
  line L13 (27.074, 16.5559) -> (27.074, -27.6401) projected
  line L14 (12.478, -27.5601) -> (27.074, -27.5601)
  line L15 (27.074, -27.5601) -> (27.074, -17.5601)
  line L16 (27.074, -17.5601) -> (12.478, -17.5601)
  line L17 (12.478, -17.5601) -> (12.478, -27.5601)
  arc A1 (24.384, -30.3301) -> (27.074, -27.6401) centre (24.384, -27.6401) ccw projected
  line L18 (26.924, 16.5559) -> (26.924, -27.6401) projected
  line L19 (27.074, -17.5601) -> (31.074, -17.5601)
  line L20 (31.074, -17.5601) -> (31.074, -27.5601)
  line L21 (31.074, -27.5601) -> (27.074, -27.5601)
  line L22 (27.074, -27.5601) -> (27.074, -17.5601)
  line L23 (31.074, -27.6401) -> (31.074, 13.9559) projected
  point P0 (0, 0)
  point P1 (27.0233, -28.1601)
  point P2 (27.074, -27.6401)
  point P3 (27.074, -27.6401)
  dimension "d22" = 1.7
  dimension "d23" = 2.4
  dimension "d24" = 1.2
  dimension "d25" = 1.25
  dimension "d26" = 3
  dimension "d27" = 1
  dimension "d28" = 0
  dimension "d29" = 0
  constraints: 24 end point, 5 parallel, 3 horizontal, 3 perpendicular, 2 collinear, 2 point on circle, 2 tangent, 1 centre point, 1 point on line
  measures "d22" distance between parallel lines of L7 L1
  measures "d23" distance between parallel lines of L6 L3
  measures "d24" distance between parallel lines of L0 L8
  measures "d25" distance between parallel lines of L9 L2
  measures "d26" radius of A0
  measures "d27" distance between parallel lines of L17 L12
  measures "d28" distance between parallel lines of L11 L16
  measures "d29" distance between parallel lines of L14 L10
extrude "power jack cutout" cut sketch "Sketch3" against normal blind 12.5 contours L12 L11 L16 L18 L14 L10 | L14 L17 L16 L12 | L18 L16 L13 L14 | L13 L19 L20 L21
sketch "Sketch6" plane through (0, 0, -1.6) normal (0, 0, -1) x (-1, 0, 0)
  arc A0 (24.384, -30.3301) -> (27.074, -27.6401) centre (24.384, -27.6401) ccw projected
  line L0 (24.384, -30.3301) -> (-24.384, -30.3301) projected
  arc A1 (-27.074, -27.6401) -> (-24.384, -30.3301) centre (-24.384, -27.6401) ccw projected
  line L1 (-27.074, -27.6401) -> (-27.074, 16.5559) projected
  arc A2 (-24.384, 19.2459) -> (-27.074, 16.5559) centre (-24.384, 16.5559) ccw projected
  line L2 (-24.384, 19.2459) -> (-19.812, 19.2459) projected
  arc A3 (-19.812, 19.2459) -> (-17.422, 21.6359) centre (-19.812, 21.6359) ccw projected
  line L3 (-17.422, 21.6359) -> (-17.422, 30.7799) projected
  arc A4 (-14.732, 33.4699) -> (-17.422, 30.7799) centre (-14.732, 30.7799) ccw projected
  line L4 (-14.732, 33.4699) -> (14.732, 33.4699) projected
  arc A5 (17.422, 30.7799) -> (14.732, 33.4699) centre (14.732, 30.7799) ccw projected
  line L5 (17.422, 30.7799) -> (17.422, 21.6359) projected
  arc A6 (17.422, 21.6359) -> (19.812, 19.2459) centre (19.812, 21.6359) ccw projected
  line L6 (19.812, 19.2459) -> (24.384, 19.2459) projected
  arc A7 (27.074, 16.5559) -> (24.384, 19.2459) centre (24.384, 16.5559) ccw projected
  line L7 (27.074, 16.5559) -> (27.074, -17.5601) projected
  line L8 (27.074, -17.5601) -> (31.074, -17.5601) projected
  line L9 (12.132, 37.4699) -> (-12.132, 37.4699) projected
  arc A8 (-12.132, 37.4699) -> (-18.922, 30.6799) centre (-12.132, 30.6799) ccw projected
  line L10 (-18.922, 30.6799) -> (-18.922, 21.7459) projected
  arc A9 (-19.922, 20.7459) -> (-18.922, 21.7459) centre (-19.922, 21.7459) ccw projected
  line L11 (-19.922, 20.7459) -> (-24.284, 20.7459) projected
  arc A10 (-24.284, 20.7459) -> (-31.074, 13.9559) centre (-24.284, 13.9559) ccw projected
  line L12 (-31.074, 13.9559) -> (-31.074, -27.6401) projected
  arc A11 (-31.074, -27.6401) -> (-24.384, -34.3301) centre (-24.384, -27.6401) ccw projected
  line L13 (-24.384, -34.3301) -> (24.384, -34.3301) projected
  arc A12 (24.384, -34.3301) -> (31.074, -27.6401) centre (24.384, -27.6401) ccw projected
  line L14 (31.074, -27.6401) -> (31.074, -27.5601) projected
  arc A13 (31.074, 13.9559) -> (24.284, 20.7459) centre (24.284, 13.9559) ccw projected
  line L15 (24.284, 20.7459) -> (19.922, 20.7459) projected
  arc A14 (18.922, 21.7459) -> (19.922, 20.7459) centre (19.922, 21.7459) ccw projected
  line L16 (18.922, 21.7459) -> (18.922, 30.6799) projected
  arc A15 (18.922, 30.6799) -> (12.132, 37.4699) centre (12.132, 30.6799) ccw projected
  line L17 (-24.88, 26.2079) -> (-21.93, 26.2079) projected
  line L18 (-18.922, 30.6799) -> (-18.922, 21.7459) projected
  line L19 (-17.422, 21.6359) -> (-17.422, 30.7799) projected
  line L20 (-18.922, 22.2079) -> (-17.422, 22.2079)
  line L21 (-17.422, 22.2079) -> (-17.422, 30.2079)
  line L22 (-17.422, 30.2079) -> (-18.922, 30.2079)
  line L23 (-18.922, 30.2079) -> (-18.922, 22.2079)
  line L24 (17.422, 30.7799) -> (17.422, 21.6359) projected
  line L25 (18.922, 21.7459) -> (18.922, 30.6799) projected
  line L26 (17.422, 22.2079) -> (18.922, 22.2079)
  line L27 (18.922, 22.2079) -> (18.922, 30.2079)
  line L28 (18.922, 30.2079) -> (17.422, 30.2079)
  line L29 (17.422, 30.2079) -> (17.422, 22.2079)
  line L30 (31.074, -27.5601) -> (27.074, -27.5601) projected
  line L31 (18.922, 30.2079) -> (18.922, 22.2079)
  line L32 (18.922, 30.6799) -> (18.922, 21.7459) projected
  line L33 (17.422, 22.2079) -> (17.422, 30.2079)
  line L34 (17.422, 30.7799) -> (17.422, 21.6359) projected
  line L35 (-18.922, 30.2079) -> (-18.922, 22.2079)
  line L36 (-18.922, 21.7459) -> (-18.922, 30.6799) projected
  line L37 (-17.422, 22.2079) -> (-17.422, 30.2079)
  line L38 (-17.422, 21.6359) -> (-17.422, 30.7799) projected
  line L39 (31.074, -17.5601) -> (31.074, 13.9559) projected
  line L40 (27.074, -27.5601) -> (27.074, -27.6401) projected
  point P0 (0, 0)
  point P1 (18.922, 30.2079)
  point P2 (17.422, 30.2079)
  point P3 (17.422, 22.2079)
  point P4 (18.922, 22.2079)
  point P5 (-17.422, 30.2079)
  point P6 (-18.922, 22.2079)
  point P7 (-17.422, 22.2079)
  dimension "d43" = 4
  dimension "d44" = 4
  constraints: 24 end point, 6 collinear, 4 parallel, 4 point on line, 2 horizontal, 2 perpendicular
  measures "d43" distance between parallel lines of L17 L20
  measures "d44" distance between parallel lines of L17 L22
extrude "rf connector cutouts" cut sketch "Sketch6" against normal blind 5.5 contours L20 L10 L22 L3 | L28 L16 L26 L5
sketch "Sketch7" plane through (0, 0, -1.6) normal (0, 0, -1) x (-1, 0, 0)
  line L0 (17.422, 30.2079) -> (18.922, 30.2079) projected
  line L1 (18.922, 30.2079) -> (18.922, 30.6799) projected
  arc A0 (18.922, 30.6799) -> (12.132, 37.4699) centre (12.132, 30.6799) ccw projected
  line L2 (12.132, 37.4699) -> (-12.132, 37.4699) projected
  arc A1 (-12.132, 37.4699) -> (-18.922, 30.6799) centre (-12.132, 30.6799) ccw projected
  line L3 (-18.922, 30.6799) -> (-18.922, 30.2079) projected
  line L4 (-18.922, 30.2079) -> (-17.422, 30.2079) projected
  line L5 (-17.422, 30.2079) -> (-17.422, 30.7799) projected
  arc A2 (-14.732, 33.4699) -> (-17.422, 30.7799) centre (-14.732, 30.7799) ccw projected
  line L6 (-14.732, 33.4699) -> (14.732, 33.4699) projected
  arc A3 (17.422, 30.7799) -> (14.732, 33.4699) centre (14.732, 30.7799) ccw projected
  line L7 (17.422, 30.7799) -> (17.422, 30.2079) projected
  line L8 (18.922, 22.2079) -> (17.422, 22.2079) projected
  line L9 (17.422, 22.2079) -> (17.422, 21.6359) projected
  arc A4 (17.422, 21.6359) -> (19.812, 19.2459) centre (19.812, 21.6359) ccw projected
  line L10 (19.812, 19.2459) -> (24.384, 19.2459) projected
  arc A5 (27.074, 16.5559) -> (24.384, 19.2459) centre (24.384, 16.5559) ccw projected
  line L11 (27.074, 16.5559) -> (27.074, -17.5601) projected
  line L12 (27.074, -17.5601) -> (31.074, -17.5601) projected
  line L13 (31.074, -27.5601) -> (27.074, -27.5601) projected
  arc A6 (24.384, -30.3301) -> (27.074, -27.6401) centre (24.384, -27.6401) ccw projected
  line L14 (24.384, -30.3301) -> (-24.384, -30.3301) projected
  arc A7 (-27.074, -27.6401) -> (-24.384, -30.3301) centre (-24.384, -27.6401) ccw projected
  line L15 (-27.074, -27.6401) -> (-27.074, 16.5559) projected
  arc A8 (-24.384, 19.2459) -> (-27.074, 16.5559) centre (-24.384, 16.5559) ccw projected
  line L16 (-24.384, 19.2459) -> (-19.812, 19.2459) projected
  arc A9 (-19.812, 19.2459) -> (-17.422, 21.6359) centre (-19.812, 21.6359) ccw projected
  line L17 (-17.422, 21.6359) -> (-17.422, 22.2079) projected
  line L18 (-17.422, 22.2079) -> (-18.922, 22.2079) projected
  line L19 (-18.922, 22.2079) -> (-18.922, 21.7459) projected
  arc A10 (-19.922, 20.7459) -> (-18.922, 21.7459) centre (-19.922, 21.7459) ccw projected
  line L20 (-19.922, 20.7459) -> (-24.284, 20.7459) projected
  arc A11 (-24.284, 20.7459) -> (-31.074, 13.9559) centre (-24.284, 13.9559) ccw projected
  line L21 (-31.074, 13.9559) -> (-31.074, -27.6401) projected
  arc A12 (-31.074, -27.6401) -> (-24.384, -34.3301) centre (-24.384, -27.6401) ccw projected
  line L22 (-24.384, -34.3301) -> (24.384, -34.3301) projected
  arc A13 (24.384, -34.3301) -> (31.074, -27.6401) centre (24.384, -27.6401) ccw projected
  line L23 (31.074, -27.6401) -> (31.074, -27.5601) projected
  arc A14 (31.074, 13.9559) -> (24.284, 20.7459) centre (24.284, 13.9559) ccw projected
  line L24 (24.284, 20.7459) -> (19.922, 20.7459) projected
  arc A15 (18.922, 21.7459) -> (19.922, 20.7459) centre (19.922, 21.7459) ccw projected
  line L25 (18.922, 21.7459) -> (18.922, 22.2079) projected
  line L26 (17.422, 22.2079) -> (17.422, 30.2079) projected
  line L27 (17.422, 22.2079) -> (18.922, 22.2079)
  line L28 (18.922, 22.2079) -> (18.922, 30.2079)
  line L29 (18.922, 30.2079) -> (17.422, 30.2079)
  line L30 (17.422, 30.2079) -> (17.422, 22.2079)
  line L31 (-18.922, 22.2079) -> (-17.422, 22.2079)
  line L32 (-17.422, 22.2079) -> (-17.422, 30.2079)
  line L33 (-17.422, 30.2079) -> (-18.922, 30.2079)
  line L34 (-18.922, 30.2079) -> (-18.922, 22.2079)
  line L35 (-27.074, -27.6401) -> (-27.074, 16.5559) projected
  line L36 (-27.074, -27.6401) -> (-27.074, -33.7654)
  arc A16 (-31.074, -27.6401) -> (-24.384, -34.3301) centre (-24.384, -27.6401) ccw projected
  arc A17 (24.384, -30.3301) -> (27.074, -27.6401) centre (24.384, -27.6401) ccw projected
  arc A18 (24.384, -34.3301) -> (31.074, -27.6401) centre (24.384, -27.6401) ccw projected
  line L37 (31.074, -27.5601) -> (12.478, -27.5601) projected
  line L38 (27.074, -27.5601) -> (27.074, -33.7654)
  line L39 (31.074, -17.5601) -> (31.074, 13.9559) projected
  line L40 (27.074, -27.5601) -> (27.074, -27.6401) projected
  point P0 (0, 0)
  point P1 (27.0233, -28.1601)
  point P2 (31.0538, -28.1601)
  point P3 (27.074, -27.6401)
  constraints: 20 end point, 4 parallel, 2 horizontal, 2 perpendicular, 2 point on circle, 2 vertical, 1 point on line, 2 other
extrude "Extrusion8" add sketch "Sketch7" along normal blind 6 contours L7 A3 L6 A2 L5 L4 L3 A1 L2 A0 L1 L0 | L8 L25 A15 L24 A14 L39 L12 L11 A5 L10 A4 L9 | L17 A9 L16 A8 L15 L36 A12 L21 A11 L20 A10 L19 L18 | L38 L13 L23 A13
ref_plane "board frontside" through (0, 0, 0) normal (0, 0, 1) x (1, 0, 0)
sketch "Sketch8" plane through (0, 0, 0) normal (0, 0, 1) x (1, 0, 0)
  line L0 (-17.422, 30.2079) -> (-18.922, 30.2079)
  line L1 (-18.922, 30.2079) -> (-18.922, 30.6799)
  arc A0 (-12.132, 37.4699) -> (-18.922, 30.6799) centre (-12.132, 30.6799) ccw
  line L2 (-12.132, 37.4699) -> (12.132, 37.4699)
  arc A1 (18.922, 30.6799) -> (12.132, 37.4699) centre (12.132, 30.6799) ccw
  line L3 (18.922, 30.6799) -> (18.922, 30.2079)
  line L4 (18.922, 30.2079) -> (17.422, 30.2079)
  line L5 (17.422, 30.2079) -> (17.422, 30.7799)
  arc A2 (17.422, 30.7799) -> (14.732, 33.4699) centre (14.732, 30.7799) ccw
  line L6 (14.732, 33.4699) -> (-14.732, 33.4699)
  arc A3 (-14.732, 33.4699) -> (-17.422, 30.7799) centre (-14.732, 30.7799) ccw
  line L7 (-17.422, 30.7799) -> (-17.422, 30.2079)
  line L8 (-19.812, 19.2459) -> (-24.384, 19.2459)
  arc A4 (-24.384, 19.2459) -> (-27.074, 16.5559) centre (-24.384, 16.5559) ccw
  line L9 (-27.074, 16.5559) -> (-27.074, -17.5601)
  line L10 (-27.074, -17.5601) -> (-31.074, -17.5601)
  line L11 (-31.074, -27.6401) -> (-31.074, -27.5601)
  arc A5 (-24.284, 20.7459) -> (-31.074, 13.9559) centre (-24.284, 13.9559) ccw
  line L12 (-24.284, 20.7459) -> (-19.922, 20.7459)
  arc A6 (-19.922, 20.7459) -> (-18.922, 21.7459) centre (-19.922, 21.7459) ccw
  line L13 (-18.922, 21.7459) -> (-18.922, 22.2079)
  line L14 (-18.922, 22.2079) -> (-17.422, 22.2079)
  line L15 (-17.422, 22.2079) -> (-17.422, 21.6359)
  arc A7 (-19.812, 19.2459) -> (-17.422, 21.6359) centre (-19.812, 21.6359) ccw
  arc A8 (27.074, -33.7654) -> (31.074, -27.6401) centre (24.384, -27.6401) ccw
  line L16 (27.074, -33.7654) -> (27.074, 16.5559)
  arc A9 (27.074, 16.5559) -> (24.384, 19.2459) centre (24.384, 16.5559) ccw
  line L17 (24.384, 19.2459) -> (19.812, 19.2459)
  arc A10 (17.422, 21.6359) -> (19.812, 19.2459) centre (19.812, 21.6359) ccw
  line L18 (17.422, 21.6359) -> (17.422, 22.2079)
  line L19 (17.422, 22.2079) -> (18.922, 22.2079)
  line L20 (18.922, 22.2079) -> (18.922, 21.7459)
  arc A11 (18.922, 21.7459) -> (19.922, 20.7459) centre (19.922, 21.7459) ccw
  line L21 (19.922, 20.7459) -> (24.284, 20.7459)
  arc A12 (31.074, 13.9559) -> (24.284, 20.7459) centre (24.284, 13.9559) ccw
  line L22 (31.074, 13.9559) -> (31.074, -27.6401)
  arc A13 (-27.074, -27.6401) -> (-24.384, -30.3301) centre (-24.384, -27.6401) ccw
  line L23 (-24.384, -30.3301) -> (24.384, -30.3301)
  arc A14 (24.384, -30.3301) -> (27.074, -27.6401) centre (24.384, -27.6401) ccw
  line L24 (27.074, -27.6401) -> (27.074, -33.7654)
  arc A15 (24.384, -34.3301) -> (27.074, -33.7654) centre (24.384, -27.6401) ccw
  line L25 (24.384, -34.3301) -> (-24.384, -34.3301)
  arc A16 (-27.074, -33.7654) -> (-24.384, -34.3301) centre (-24.384, -27.6401) ccw
  line L26 (-27.074, -17.5601) -> (-31.074, -17.5601)
  line L27 (-27.074, -17.5601) -> (-25.574, -17.5601)
  line L28 (-25.574, -17.5601) -> (-25.574, -2.5601)
  line L29 (-25.574, -2.5601) -> (-27.074, -2.5601)
  line L30 (-27.074, -2.5601) -> (-27.074, -17.5601)
  line L31 (14.732, 33.4699) -> (-14.732, 33.4699)
  line L32 (-12.422, 33.4699) -> (12.422, 33.4699)
  line L33 (12.422, 33.4699) -> (12.422, 31.9699)
  line L34 (12.422, 31.9699) -> (-12.422, 31.9699)
  line L35 (-12.422, 31.9699) -> (-12.422, 33.4699)
  line L36 (27.074, -33.7654) -> (27.074, 16.5559)
  line L37 (27.074, 7.9459) -> (25.574, 7.9459)
  line L38 (25.574, 7.9459) -> (25.574, 16.5559)
  line L39 (25.574, 16.5559) -> (27.074, 16.5559)
  line L40 (27.074, 16.5559) -> (27.074, 7.9459)
  line L41 (26.45, 6.4459) -> (-13.75, 6.4459)
  line L42 (-13.75, -6.3541) -> (26.45, -6.3541)
  line L43 (27.074, -7.8541) -> (25.574, -7.8541)
  line L44 (25.574, -7.8541) -> (25.574, -17.8541)
  line L45 (25.574, -17.8541) -> (27.074, -17.8541)
  line L46 (27.074, -17.8541) -> (27.074, -7.8541)
  line L47 (-24.384, -30.3301) -> (24.384, -30.3301)
  line L48 (-24.384, -30.3301) -> (-4.384, -30.3301)
  line L49 (-4.384, -30.3301) -> (-4.384, -28.8301)
  line L50 (-4.384, -28.8301) -> (-24.384, -28.8301)
  line L51 (-24.384, -28.8301) -> (-24.384, -30.3301)
  line L52 (4.616, -30.3301) -> (11.074, -30.3301)
  line L53 (11.074, -30.3301) -> (11.074, -28.8301)
  line L54 (11.074, -28.8301) -> (4.616, -28.8301)
  line L55 (4.616, -28.8301) -> (4.616, -30.3301)
  line L56 (-27.074, 16.5559) -> (-27.074, -17.5601)
  line L57 (-27.074, 6.5559) -> (-25.574, 6.5559)
  line L58 (-25.574, 6.5559) -> (-25.574, 16.5559)
  line L59 (-25.574, 16.5559) -> (-27.074, 16.5559)
  line L60 (-27.074, 16.5559) -> (-27.074, 6.5559)
  line L61 (24.384, 19.2459) -> (19.812, 19.2459)
  line L62 (19.812, 19.2459) -> (24.384, 19.2459)
  line L63 (24.384, 19.2459) -> (24.384, 17.7459)
  line L64 (24.384, 17.7459) -> (19.812, 17.7459)
  line L65 (19.812, 17.7459) -> (19.812, 19.2459)
  line L66 (-19.812, 19.2459) -> (-24.384, 19.2459)
  line L67 (-24.384, 19.2459) -> (-19.812, 19.2459)
  line L68 (-19.812, 19.2459) -> (-19.812, 17.7459)
  line L69 (-19.812, 17.7459) -> (-24.384, 17.7459)
  line L70 (-24.384, 17.7459) -> (-24.384, 19.2459)
  line L71 (-25.773, -8.637) -> (-25.773, -11.0832)
  line L72 (-25.773, -11.0832) -> (-25.2261, -11.6301)
  line L73 (-25.2261, -8.0901) -> (-25.773, -8.637)
  line L74 (-17.924, -28.8301) -> (-15.924, -28.8301)
  line L75 (-15.924, -28.8301) -> (-15.924, -30.3301)
  line L76 (-15.924, -30.3301) -> (-17.924, -30.3301)
  line L77 (-17.924, -30.3301) -> (-17.924, -28.8301)
  line L78 (-17.924, -28.8301) -> (-19.924, -28.8301)
  line L79 (-19.924, -28.8301) -> (-19.924, -30.3301)
  line L80 (-19.924, -30.3301) -> (-17.924, -30.3301)
  line L81 (-17.924, -30.3301) -> (-17.924, -28.8301)
  line L82 (-26.924, 16.5559) -> (-26.924, -27.6401)
  line L83 (-27.074, -33.7654) -> (-27.074, -27.6401)
  line L84 (-27.074, -27.5601) -> (-27.074, -33.7654)
  arc A17 (-31.074, -27.6401) -> (-27.074, -33.7654) centre (-24.384, -27.6401) ccw
  line L85 (-31.074, -27.5601) -> (-27.074, -27.5601)
  line L86 (-31.074, -17.5601) -> (-31.074, 13.9559)
  point P0 (0, 0)
  point P1 (-27.074, -2.5601)
  point P2 (-25.574, -11.2822)
  point P3 (-25.574, -8.438)
extrude "board support standoffs" add sketch "Sketch8" along normal up to surface (5.9 mm away) contours L6 L33 L34 L35 | L68 L69 L70 L8 | L59 L82 L57 L9 | L59 L58 L57 L82 | L29 L82 L27 L9 | L29 L28 L73 L71 L72 L27 L82 | L51 L50 L79 L23 | L45 L44 L43 L16 | L75 L50 L49 L23 | L23 L55 L54 L53 | L37 L38 L39 L16 | L63 L64 L65 L17